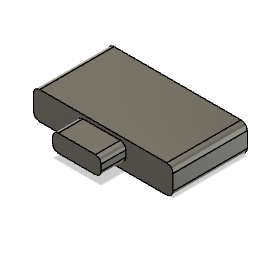
LED retaining Peg v1 (Autodesk Fusion 360 design; units mm, degrees)
Autodesk Fusion 360 part; units mm, degrees
sketch "Sketch1" plane through (0, 0, 0) normal (0, 1, 0) x (1, 0, 0)
  line L0 (14.75, 62.5) -> (-14.75, 62.5)
  line L1 (-14.75, 62.5) -> (-14.75, -62.5)
  line L2 (-14.75, -62.5) -> (14.75, -62.5)
  line L3 (14.75, -62.5) -> (14.75, 62.5)
  line L4 (14.75, 62.5) -> (-14.75, -62.5) construction
  line L5 (-14.75, 62.5) -> (14.75, -62.5) construction
  dimension "d1" = 29.5
  dimension "d4" = 125
  constraint perpendicular L0 L1
  constraint parallel L0 L2
  constraint parallel L1 L3
  constraint horizontal L0
  constraint coincident L4 origin
  constraint coincident L5 origin
  measures "d1" distance of L1.end L2.end
  measures "d4" distance of L0.end L1.end
extrude "Extrude1" add sketch "Sketch1" along normal blind 25 makes body 1
sketch "Sketch2" plane through (14.75, 0, 0) normal (1, 0, 0) x (0, 0, -1)
  line L0 (-62.5, 0) -> (62.5, 0)
  line L1 (62.5, 25) -> (-62.5, 25)
  line L2 (-62.5, 25) -> (-62.5, 0)
  line L3 (-57.5, 0) -> (-41.5, 0)
  line L4 (-41.5, 0) -> (-41.5, 22)
  line L5 (-41.5, 22) -> (-57.5, 22)
  line L6 (-57.5, 22) -> (-57.5, 0)
  dimension "d5" = 16
  dimension "d6" = 5
  dimension "d70" = 3
  constraint horizontal L3
  constraint vertical L4
  constraint horizontal L5
  constraint vertical L6
  constraint coincident L0 L3.start
  measures "d5" distance of L4.end L5.end
  measures "d6" distance of L2 L6
  measures "d70" distance of L1 L5
sketch "Sketch3" plane through (-14.75, 0, 0) normal (-1, 0, 0) x (0, 0, 1)
  line L0 (62.5, 0) -> (62.5, 25)
  line L1 (62.5, 25) -> (-62.5, 25)
  line L2 (-62.5, 25) -> (-62.5, 0)
  line L3 (-62.5, 0) -> (62.5, 0)
  line L4 (-57.5, 0) -> (54.5, 0)
  line L5 (54.5, 0) -> (54.5, 17)
  line L6 (54.5, 17) -> (-57.5, 17)
  line L7 (-57.5, 17) -> (-57.5, 0)
  dimension "d51" = 5
  dimension "d69" = 8
  dimension "d93" = 112
  constraint horizontal L4
  constraint vertical L5
  constraint horizontal L6
  constraint vertical L7
  constraint collinear L3 L4
  measures "d51" distance of L2 L7
  measures "d69" distance of L1 L6
  measures "d93" distance of L5 L7
extrude "Extrude3" cut sketch "Sketch3" against normal blind 26 contours L3 L4 L5 L6 L7 bodies 1
sketch "Sketch4" plane through (-14.75, 0, 0) normal (-1, 0, 0) x (0, 0, 1)
  line L0 (54.5, 17) -> (54.5, 0)
  line L1 (54.5, 0) -> (62.5, 0)
  line L2 (62.5, 0) -> (62.5, 25)
  line L3 (62.5, 25) -> (-62.5, 25)
  line L4 (-62.5, 25) -> (-62.5, 0)
  line L5 (-62.5, 0) -> (-57.5, 0)
  line L6 (-57.5, 17) -> (54.5, 17)
  line L7 (-54.0622, 25) -> (-48, 21.5)
  line L8 (-48, 21.5) -> (37, 21.5)
  line L9 (37, 21.5) -> (43.0622, 25)
  line L10 (-57.5, 0) -> (-57.5, 17)
  dimension "d16" = 3.5
  dimension "d44" = 150
  dimension "d45" = 150
  dimension "d46" = 85
  dimension "d116" = 14.5
  constraint coincident L3 L7.start
  constraint parallel L3 L8
  constraint coincident L3 L9.end
  measures "d16" vertical distance of L7.start L7.end
  measures "d44" angle of L7 L8
  measures "d45" angle of L8 L9
  measures "d46" distance of L7.end L8.end
  measures "d116" distance of L4 L7.end
extrude "Extrude4" cut sketch "Sketch4" against normal through all contours L3 L7 L8 L9 bodies 1
sketch "Sketch5" plane through (-14.75, 0, 0) normal (-1, 0, 0) x (0, 0, 1)
  line L0 (43.0622, 25) -> (37, 21.5)
  line L1 (37, 21.5) -> (-48, 21.5)
  line L2 (-48, 21.5) -> (-54.0622, 25)
  line L3 (-62.5, 25) -> (-62.5, 0)
  line L4 (-62.5, 0) -> (-57.5, 0)
  line L5 (-57.5, 17) -> (54.5, 17)
  line L6 (54.5, 17) -> (54.5, 0)
  line L7 (54.5, 0) -> (62.5, 0)
  line L8 (-53, 21.5) -> (50.5, 21.5)
  line L9 (50.5, 21.5) -> (50.5, 18.55)
  line L10 (50.5, 18.55) -> (-53, 18.55)
  line L11 (-53, 18.55) -> (-53, 21.5)
  line L12 (-57.5, 0) -> (-57.5, 17)
  line L13 (62.5, 0) -> (62.5, 25)
  line L14 (-54.0622, 25) -> (-62.5, 25)
  line L15 (62.5, 25) -> (43.0622, 25)
  dimension "d22" = 2.95
  dimension "d48" = 13.5
  dimension "d107" = 5
  constraint horizontal L8
  constraint vertical L9
  constraint horizontal L10
  constraint vertical L11
  constraint collinear L1 L8
  measures "d22" distance of L8.start L10.end
  measures "d48" distance of L0.end L8.end
  measures "d107" distance of L1.end L8.start
extrude "Extrude5" cut sketch "Sketch5" against normal blind 26 contours L1 L8 L9 L10 L11 bodies 1
sketch "Sketch14" plane through (-14.75, 0, 0) normal (-1, 0, 0) x (0, 0, 1)
  line L0 (37, 21.5) -> (50.5, 21.5)
  line L1 (50.5, 21.5) -> (50.5, 18.55)
  line L2 (50.5, 18.55) -> (-53, 18.55)
  line L3 (-53, 18.55) -> (-53, 21.5)
  line L4 (-48, 21.5) -> (-54.0622, 25)
  line L5 (-54.0622, 25) -> (-62.5, 25)
  line L6 (-62.5, 25) -> (-62.5, 0)
  line L7 (-62.5, 0) -> (-57.5, 0)
  line L8 (-57.5, 0) -> (-57.5, 17)
  line L9 (-57.5, 17) -> (54.5, 17)
  line L10 (54.5, 17) -> (54.5, 0)
  line L11 (54.5, 0) -> (62.5, 0)
  line L12 (62.5, 0) -> (62.5, 25)
  line L13 (62.5, 25) -> (43.0622, 25)
  line L14 (43.0622, 25) -> (37, 21.5)
  line L15 (-53, 21.5) -> (50.5, 21.5)
  line L16 (50.5, 21.5) -> (50.5, 21.75)
  line L17 (50.5, 21.75) -> (-53, 21.75)
  line L18 (-53, 21.75) -> (-53, 21.5)
  line L19 (-53, 21.5) -> (-48, 21.5)
  dimension "d90" = 0.25
  constraint horizontal L15
  constraint vertical L16
  constraint horizontal L17
  constraint vertical L18
  constraint coincident L3.end L15.start
  constraint collinear L1 L16
  measures "d90" distance of L15 L17
extrude "Extrude14" cut sketch "Sketch14" against normal up to surface (26 mm away) contours L0 L14 L15 L16 L17 | L4 L15 L17 L18 L19 bodies 1
ref_plane "WorkPlane1" through (0, 12.5, 0) normal (0, 0, -1) x (-1, 0, 0)
sketch "Sketch6" plane through (0, 0, -62.5) normal (0, 0, -1) x (-1, 0, 0)
  line L0 (-14.75, 0) -> (14.75, 0)
  line L1 (14.75, 0) -> (14.75, 25)
  line L2 (-14.75, 25) -> (-14.75, 0)
  line L3 (14.75, 25) -> (-14.75, 25)
  line L4 (14.75, 17) -> (14.75, 8)
  line L5 (14.75, 8) -> (17.75, 8)
  line L6 (17.75, 8) -> (17.75, 17)
  line L7 (17.75, 17) -> (14.75, 17)
  line L8 (17.75, 12.5) -> (14.75, 12.5) construction
  dimension "d52" = 8
  dimension "d53" = 8
  dimension "d54" = 3
  constraint coincident L1 L4.start
  constraint coincident L1 L4.end
  constraint perpendicular L3 L4
  constraint parallel L1 L6
  constraint midpoint L6 L8.start
  constraint midpoint L4 L8.end
  constraint horizontal L8
  constraint horizontal L7
  measures "d52" distance of L0 L4.end
  measures "d53" distance of L3 L4.start
  measures "d54" distance of L4 L6
sketch "Sketch7" plane through (0, 0, -62.5) normal (0, 0, -1) x (-1, 0, 0)
  line L0 (14.75, 0) -> (-14.75, 0)
  line L1 (-14.75, 0) -> (-14.75, 25)
  line L2 (-14.75, 17) -> (-14.75, 8)
  line L3 (-14.75, 8) -> (-11.75, 8)
  line L4 (-14.75, 17) -> (-11.75, 17)
  line L5 (-11.75, 17) -> (-11.75, 8)
  line L6 (-11.75, 12.5) -> (-14.75, 12.5) construction
  dimension "d56" = 8
  dimension "d57" = 8
  dimension "d58" = 3
  constraint coincident L1 L2.start
  constraint coincident L1 L2.end
  constraint midpoint L5 L6.start
  constraint midpoint L2 L6.end
  constraint horizontal L6
  constraint horizontal L4
  measures "d56" distance of L0.end L2.end
  measures "d57" distance of L1.end L2.start
  measures "d58" distance of L2 L5
extrude "Extrude6" add sketch "Sketch6" against normal blind 5 contours L1 L4 L5 L6 L7 bodies 1
extrude "Extrude7" cut sketch "Sketch7" against normal blind 5.5 bodies 1
mirror "Mirror1" about plane through (0, 12.5, 0) normal (0, 0, -1) of "Extrude6", "Extrude7"
sketch "Sketch10" plane through (0, 0, -62.5) normal (0, 0, -1) x (-1, 0, 0)
  line L0 (-11.75, 8) -> (-14.75, 8)
  line L1 (-14.75, 8) -> (-14.75, 0)
  line L2 (-14.75, 0) -> (14.75, 0)
  line L3 (14.75, 0) -> (14.75, 8)
  line L4 (14.75, 8) -> (17.75, 8)
  line L5 (17.75, 8) -> (17.75, 17)
  line L6 (17.75, 17) -> (14.75, 17)
  line L7 (14.75, 17) -> (14.75, 25)
  line L8 (14.75, 25) -> (-14.75, 25)
  line L9 (-14.75, 25) -> (-14.75, 17)
  line L10 (-14.75, 17) -> (-11.75, 17)
  line L11 (-11.75, 17) -> (-11.75, 8)
  circle A0 centre (1.75, 8) radius 2
  line L12 (14.75, 17) -> (-11.25, 17)
  line L13 (1.75, 8) -> (1.75, 17) construction
  dimension "d60" = 4
  dimension "d61" = 8
  constraint coincident A0.centre L13.start
  constraint midpoint L12 L13.end
  constraint perpendicular L12 L13
  measures "d60" diameter of A0
  measures "d61" distance of L2 A0.centre
extrude "Extrude10" cut sketch "Sketch10" against normal blind 5 contours A0 bodies 1
sketch "Sketch12" plane through (14.75, 0, 0) normal (1, 0, 0) x (0, 0, -1)
  line L0 (-62.5, 17) -> (-57, 17)
  line L1 (-62.5, 0) -> (62.5, 0)
  line L2 (62.5, 0) -> (62.5, 8)
  line L3 (62.5, 8) -> (57, 8)
  line L4 (57, 8) -> (57, 17)
  line L5 (57, 17) -> (62.5, 17)
  line L6 (62.5, 17) -> (62.5, 25)
  line L7 (62.5, 25) -> (54.0622, 25)
  line L8 (54.0622, 25) -> (48, 21.5)
  line L9 (48, 21.5) -> (-37, 21.5)
  line L10 (-37, 21.5) -> (-43.0622, 25)
  line L11 (-43.0622, 25) -> (-62.5, 25)
  line L12 (-62.5, 8) -> (-62.5, 0)
  line L13 (-41.5, 18.5) -> (-45, 22)
  line L14 (-57, 17) -> (-57, 8)
  line L15 (-57, 8) -> (-62.5, 8)
  line L16 (-62.5, 25) -> (-62.5, 17)
sketch "Sketch13" plane through (0, 0, 62.5) normal (0, 0, 1) x (1, 0, 0)
  line L0 (14.75, 8) -> (11.75, 8)
  line L1 (11.75, 8) -> (11.75, 17)
  line L2 (11.75, 17) -> (14.75, 17)
  line L3 (14.75, 17) -> (14.75, 25)
  line L4 (14.75, 25) -> (-14.75, 25)
  line L5 (-14.75, 25) -> (-14.75, 17)
  line L6 (-14.75, 17) -> (-17.75, 17)
  line L7 (-17.75, 17) -> (-17.75, 8)
  line L8 (-17.75, 8) -> (-14.75, 8)
  line L9 (-14.75, 8) -> (-14.75, 0)
  line L10 (-14.75, 0) -> (14.75, 0)
  line L11 (14.75, 0) -> (14.75, 8)
  line L12 (14.75, 17.4) -> (11.35, 17.4)
  line L13 (11.35, 17.4) -> (11.35, 7.6)
  line L14 (11.35, 7.6) -> (14.75, 7.6)
  dimension "d83" = 0.4
  dimension "d84" = 0.4
  dimension "d85" = 0.4
  constraint coincident L3 L12.start
  constraint parallel L1 L13
  constraint coincident L11 L14.end
  constraint parallel L0 L14
  constraint parallel L2 L12
  measures "d83" distance of L2 L12
  measures "d84" distance of L0 L14
  measures "d85" distance of L1 L13
extrude "Extrude13" cut sketch "Sketch13" against normal blind 5.5 contours L0 L1 L2 L3 L11 L12 L13 L14 bodies 1
mirror "Mirror2" about plane through (0, 0, 0) normal (0, 0, 1) of "Extrude13"
sketch "Sketch15" plane through (0, 17, 0) normal (0, -1, 0) x (1, 0, 0)
  line L0 (-14.75, 54.5) -> (-14.75, -57.5)
  line L1 (-14.75, -57.5) -> (11.25, -57.5)
  line L2 (11.25, -57.5) -> (11.25, 54.5)
  line L3 (11.25, 54.5) -> (-14.75, 54.5)
  line L4 (11.25, 50.5) -> (-14.75, 50.5) construction
  line L5 (-4.75, 51.5) -> (1.25, 51.5)
  line L6 (1.25, 51.5) -> (1.25, 45.5)
  line L7 (1.25, 45.5) -> (-4.75, 45.5)
  line L8 (-4.75, 45.5) -> (-4.75, 51.5)
  line L9 (-4.75, 50) -> (-6.95, 50)
  line L10 (-6.95, 50) -> (-6.95, 47)
  line L11 (-6.95, 47) -> (-4.75, 47)
  line L12 (-4.75, 47) -> (-4.75, 50)
  line L13 (1.25, 50) -> (3.45, 50)
  line L14 (3.45, 50) -> (3.45, 47)
  line L15 (3.45, 47) -> (1.25, 47)
  line L16 (1.25, 47) -> (1.25, 50)
  line L17 (-14.75, 50.5) -> (11.25, 50.5)
  line L18 (-1.75, 50.5) -> (-1.75, 51.5) construction
  dimension "d94" = 6
  dimension "d95" = 6
  dimension "d96" = 2.2
  dimension "d97" = 3
  dimension "d118" = 1
  constraint horizontal L5
  constraint vertical L6
  constraint horizontal L7
  constraint vertical L8
  constraint horizontal L9
  constraint vertical L10
  constraint horizontal L11
  constraint vertical L12
  constraint coincident L8 L9.start
  constraint horizontal L13
  constraint vertical L14
  constraint horizontal L15
  constraint vertical L16
  constraint coincident L6 L13.start
  constraint midpoint L8 L12
  constraint midpoint L6 L16
  constraint equal L9 L13
  constraint equal L10 L14
  constraint midpoint L4 L18.start
  constraint midpoint L5 L18.end
  constraint vertical L18
  measures "d94" distance of L5.start L5.end
  measures "d95" distance of L5.start L7.end
  measures "d96" distance of L9.start L9.end
  measures "d97" distance of L9.end L10.end
  measures "d118" distance of L4 L5
extrude "Extrude15" cut sketch "Sketch15" against normal up to surface (4.75 mm away) contours L6 L7 L8 L12 L16 L17 | L5 L6 L8 L17 | L8 L9 L10 L11 L12 | L6 L13 L14 L15 L16 bodies 1
sketch "Sketch17" plane through (-14.75, 0, 0) normal (-1, 0, 0) x (0, 0, 1)
  line L0 (57.5, 17) -> (62.5, 17)
  line L1 (62.5, 17) -> (62.5, 25)
  line L2 (62.5, 25) -> (43.0622, 25)
  line L3 (43.0622, 25) -> (37.433, 21.75)
  line L4 (37.433, 21.75) -> (50.5, 21.75)
  line L5 (50.5, 21.75) -> (50.5, 18.55)
  line L6 (50.5, 18.55) -> (-53, 18.55)
  line L7 (-53, 18.55) -> (-53, 21.75)
  line L8 (-53, 21.75) -> (-48.433, 21.75)
  line L9 (-48.433, 21.75) -> (-54.0622, 25)
  line L10 (-54.0622, 25) -> (-62.5, 25)
  line L11 (-62.5, 25) -> (-62.5, 17)
  line L12 (-62.5, 17) -> (-57.5, 17)
  line L13 (-57.5, 17) -> (54.5, 17)
  line L14 (54.5, 17) -> (54.5, 0)
  line L15 (-57.9, 23.5125) -> (54.9, 23.5125)
  line L16 (54.9, 23.5125) -> (54.9, 20.9313)
  line L17 (54.9, 20.9313) -> (-57.9, 20.9313)
  line L18 (-57.9, 20.9313) -> (-57.9, 23.5125)
  line L19 (62.5, 8) -> (57.5, 8)
  line L20 (57.5, 8) -> (57.5, 17)
  line L21 (54.5, 0) -> (62.5, 0)
  line L22 (62.5, 0) -> (62.5, 8)
  dimension "d109" = 2.3813
  dimension "d110" = 2.5812
  dimension "d111" = 4.6
  dimension "d115" = 112.8
  constraint horizontal L15
  constraint vertical L16
  constraint horizontal L17
  constraint vertical L18
  constraint coincident L16.end L17.start
  measures "d109" distance of L6 L17
  measures "d110" distance of L15.start L17.end
  measures "d111" distance of L11 L18
  measures "d115" distance of L15.start L15.end
extrude "Extrude17" cut sketch "Sketch17" against normal blind 30 contours L3 L4 L5 L15 L16 L17 | L3 L4 L5 L7 L8 L9 L15 L17 | L7 L8 L9 L15 L17 L18 bodies 1
sketch "Sketch18" plane through (11.25, 0, 0) normal (-1, 0, 0) x (0, 0, 1)
  line L0 (-57.5, 17) -> (-57.5, 0)
  line L1 (-57.5, 0) -> (54.5, 0)
  line L2 (54.5, 0) -> (54.5, 17)
  line L3 (54.5, 17) -> (-57.5, 17)
  line L4 (42.5, 17) -> (54.5, 17)
  line L5 (54.5, 17) -> (54.5, 0)
  line L6 (54.5, 0) -> (42.5, 0)
  line L7 (42.5, 0) -> (42.5, 17)
  line L8 (50, 17) -> (47, 17)
  line L9 (48.5, 17) -> (48.5, 0) construction
  dimension "d117" = 12
  constraint horizontal L4
  constraint vertical L5
  constraint horizontal L6
  constraint vertical L7
  constraint coincident L1 L2.start
  constraint coincident L3 L4.start
  constraint midpoint L6 L9.end
  constraint coincident L8 L9.start
  constraint vertical L9
  constraint midpoint L8 L9.start
  measures "d117" distance of L1.end L6.end
extrude "Extrude18" cut sketch "Sketch18" against normal through all contours L1 L2 L3 L4 L5 L6 L7 L8 bodies 1
fillet "Fillet5" radius 1 4 edges at (-6.95, 17.775, 50) (-6.95, 17.775, 47) (3.45, 17.775, 47) (3.45, 17.775, 50) on bodies 1
sketch "Sketch19" plane through (11.25, 0, 0) normal (-1, 0, 0) x (0, 0, 1)
  line L0 (50.5, 20.9313) -> (-53, 20.9313)
  line L1 (-53, 20.9313) -> (-53, 18.55)
  line L2 (-53, 18.55) -> (50.5, 18.55)
  line L3 (50.5, 18.55) -> (50.5, 20.9313)
  line L4 (-53, 20.9313) -> (50.5, 20.9313)
  line L5 (50.5, 20.9313) -> (50.5, 20.8813)
  line L6 (50.5, 20.8813) -> (-53, 20.8813)
  line L7 (-53, 20.8813) -> (-53, 20.9313)
  constraint horizontal L4
  constraint vertical L5
  constraint horizontal L6
  constraint vertical L7
  constraint coincident L3 L5.end
  constraint coincident L0.end L1.start
extrude "Extrude19" cut sketch "Sketch19" against normal through all contours L0 L1 L3 L4 L5 L6 L7 bodies 1
sketch "Sketch20" plane through (0, 17, 0) normal (0, -1, 0) x (1, 0, 0)
  line L0 (1.25, 50) -> (2.45, 50)
  arc A0 (3.45, 49) -> (2.45, 50) centre (2.45, 49) ccw
  line L1 (3.45, 49) -> (3.45, 48)
  arc A1 (2.45, 47) -> (3.45, 48) centre (2.45, 48) ccw
  line L2 (2.45, 47) -> (1.25, 47)
  line L3 (1.25, 47) -> (1.25, 45.5)
  line L4 (1.25, 45.5) -> (-4.75, 45.5)
  line L5 (-4.75, 45.5) -> (-4.75, 47)
  line L6 (-4.75, 47) -> (-5.95, 47)
  arc A2 (-6.95, 48) -> (-5.95, 47) centre (-5.95, 48) ccw
  line L7 (-6.95, 48) -> (-6.95, 49)
  arc A3 (-5.95, 50) -> (-6.95, 49) centre (-5.95, 49) ccw
  line L8 (-5.95, 50) -> (-4.75, 50)
  line L9 (-4.75, 50) -> (-4.75, 51.5)
  line L10 (-4.75, 51.5) -> (1.25, 51.5)
  line L11 (1.25, 51.5) -> (1.25, 50)
  line L12 (-14.75, 54.5) -> (-14.75, -57.5)
  line L13 (-14.75, -57.5) -> (11.25, -57.5)
  line L14 (11.25, -57.5) -> (11.25, 42.5)
  line L15 (11.25, 42.5) -> (14.75, 42.5)
  line L16 (14.75, 42.5) -> (14.75, 54.5)
  line L17 (14.75, 54.5) -> (-14.75, 54.5)
  line L18 (11.25, 42.5) -> (-14.75, 42.5)
  constraint coincident L14.end L15.start
  constraint coincident L12 L18.end
  constraint perpendicular L12 L18
extrude "Extrude20" add sketch "Sketch20" along normal blind 0.5 contours L12 L15 L16 L17 L18 bodies 1
sketch "Sketch21" plane through (14.75, 0, 0) normal (1, 0, 0) x (0, 0, -1)
  line L0 (-50.5, 20.8813) -> (-50.5, 20.9313)
  line L1 (-50.5, 20.9313) -> (-54.9, 20.9313)
  line L2 (-54.9, 20.9313) -> (-54.9, 23.5125)
  line L3 (-54.9, 23.5125) -> (-40.4858, 23.5125)
  line L4 (-40.4858, 23.5125) -> (-43.0622, 25)
  line L5 (-43.0622, 25) -> (-62.5, 25)
  line L6 (-62.5, 25) -> (-62.5, 17.4)
  line L7 (-62.5, 17.4) -> (-57, 17.4)
  line L8 (-57, 17.4) -> (-57, 7.6)
  line L9 (-57, 7.6) -> (-62.5, 7.6)
  line L10 (-62.5, 7.6) -> (-62.5, 0)
  line L11 (-62.5, 0) -> (-54.5, 0)
  line L12 (-54.5, 0) -> (-54.5, 16.5)
  line L13 (-54.5, 16.5) -> (-42.5, 16.5)
  line L14 (-42.5, 16.5) -> (-42.5, 0)
  line L15 (-42.5, 0) -> (62.5, 0)
  line L16 (62.5, 0) -> (62.5, 7.6)
  line L17 (62.5, 7.6) -> (57, 7.6)
  line L18 (57, 7.6) -> (57, 17.4)
  line L19 (57, 17.4) -> (62.5, 17.4)
  line L20 (62.5, 17.4) -> (62.5, 25)
  line L21 (62.5, 25) -> (54.0622, 25)
  line L22 (54.0622, 25) -> (51.4858, 23.5125)
  line L23 (51.4858, 23.5125) -> (57.9, 23.5125)
  line L24 (57.9, 23.5125) -> (57.9, 20.9313)
  line L25 (57.9, 20.9313) -> (53, 20.9313)
  line L26 (53, 20.9313) -> (53, 20.8813)
  line L27 (53, 20.8813) -> (-50.5, 20.8813)
  line L28 (-54.5, 14.5) -> (-52.5, 16.5)
  line L29 (-42.5, 14.5) -> (-44.5, 16.5)
  dimension "d125" = 2
  dimension "d126" = 2
  dimension "d127" = 2
  constraint coincident L12 L28.start
  constraint coincident L13 L28.end
  constraint coincident L14 L29.start
  constraint coincident L13 L29.end
  constraint perpendicular L28 L29
  measures "d125" distance of L12.end L28.end
  measures "d126" distance of L14 L29.end
  measures "d127" distance of L13 L29.start
extrude "Extrude21" add sketch "Sketch21" against normal up to surface (3.5 mm away) contours L12 L13 L28 | L13 L14 L29 bodies 1
sketch "Sketch22" plane through (0, 0, 54.5) normal (0, 0, -1) x (-1, 0, 0)
  line L0 (-11.25, 14.5) -> (-14.75, 14.5)
  line L1 (-14.75, 14.5) -> (-14.75, 0)
  line L2 (-14.75, 0) -> (14.75, 0)
  line L3 (14.75, 0) -> (14.75, 16.5)
  line L4 (14.75, 16.5) -> (-11.25, 16.5)
  line L5 (-11.25, 16.5) -> (-11.25, 14.5)
  line L6 (-2.25, 15.5) -> (5.75, 15.5)
  line L7 (5.75, 15.5) -> (5.75, 12.5)
  line L8 (5.75, 12.5) -> (-2.25, 12.5)
  line L9 (-2.25, 12.5) -> (-2.25, 15.5)
  line L10 (1.75, 16.5) -> (1.75, 15.5) construction
  dimension "d130" = 3
  dimension "d131" = 8
  dimension "d132" = 1
  constraint horizontal L6
  constraint vertical L7
  constraint horizontal L8
  constraint vertical L9
  constraint midpoint L4 L10.start
  constraint midpoint L6 L10.end
  constraint vertical L10
  measures "d130" distance of L6.start L8.end
  measures "d131" distance of L7.end L8.end
  measures "d132" distance of L4 L6
extrude "Extrude22" cut sketch "Sketch22" against normal blind 4 contours L6 L7 L8 L9 bodies 1
fillet "Fillet6" radius 1 4 edges at (2.25, 15.5, 56.5) (2.25, 12.5, 56.5) (-5.75, 12.5, 56.5) (-5.75, 15.5, 56.5) on bodies 1
sketch "Sketch23" plane through (0, 16.5, 0) normal (0, -1, 0) x (1, 0, 0)
  line L0 (11.25, 44.5) -> (14.75, 44.5)
  line L1 (14.75, 44.5) -> (14.75, 52.5)
  line L2 (14.75, 52.5) -> (11.25, 52.5)
  line L3 (11.25, 52.5) -> (11.25, 54.5)
  line L4 (11.25, 54.5) -> (-14.75, 54.5)
  line L5 (-14.75, 54.5) -> (-14.75, 42.5)
  line L6 (-14.75, 42.5) -> (11.25, 42.5)
  line L7 (11.25, 42.5) -> (11.25, 44.5)
  arc A0 (-5.95, 50) -> (-6.95, 49) centre (-5.95, 49) ccw
  line L8 (-5.95, 50) -> (-4.75, 50)
  line L9 (-4.75, 50) -> (-4.75, 51.5)
  line L10 (-4.75, 51.5) -> (1.25, 51.5)
  line L11 (1.25, 51.5) -> (1.25, 50)
  line L12 (1.25, 50) -> (2.45, 50)
  arc A1 (3.45, 49) -> (2.45, 50) centre (2.45, 49) ccw
  line L13 (3.45, 49) -> (3.45, 48)
  arc A2 (2.45, 47) -> (3.45, 48) centre (2.45, 48) ccw
  line L14 (2.45, 47) -> (1.25, 47)
  line L15 (1.25, 47) -> (1.25, 45.5)
  line L16 (1.25, 45.5) -> (-4.75, 45.5)
  line L17 (-4.75, 45.5) -> (-4.75, 47)
  line L18 (-4.75, 47) -> (-5.95, 47)
  arc A3 (-6.95, 48) -> (-5.95, 47) centre (-5.95, 48) ccw
  line L19 (-6.95, 48) -> (-6.95, 49)
  line L20 (-14.75, 54.5) -> (11.25, 54.5)
  line L21 (11.25, 54.5) -> (11.25, 42.5)
  line L22 (11.25, 42.5) -> (-14.75, 42.5)
  line L23 (-14.75, 42.5) -> (-14.75, 54.5)
  line L24 (11.25, 54.5) -> (9.75, 54.5) construction
  line L25 (9.75, 54.5) -> (9.75, 42.5)
  line L26 (9.75, 42.5) -> (11.25, 42.5) construction
  line L27 (11.25, 42.5) -> (11.25, 54.5) construction
  line L28 (-14.75, 54.5) -> (-12.75, 54.5) construction
  line L29 (-12.75, 54.5) -> (-12.75, 42.5)
  line L30 (-12.75, 42.5) -> (-14.75, 42.5) construction
  line L31 (-14.75, 42.5) -> (-14.75, 54.5) construction
  dimension "d139" = 1.5
  dimension "d140" = 2
  dimension "d141" = 12
  constraint horizontal L20
  constraint vertical L21
  constraint horizontal L22
  constraint vertical L23
  constraint coincident L6.end L7.start
  constraint coincident L4.end L5.start
  constraint horizontal L24
  constraint vertical L25
  constraint horizontal L26
  constraint vertical L27
  constraint horizontal L28
  constraint vertical L29
  constraint horizontal L30
  constraint vertical L31
  measures "d139" distance of L3.end L24.end
  measures "d140" distance of L4.end L28.end
  measures "d141" distance of L4.end L5.end
sketch "Sketch24" plane through (0, 0, 54.5) normal (0, 0, -1) x (-1, 0, 0)
  line L0 (5.75, 14.5) -> (5.75, 13.5)
  arc A0 (4.75, 12.5) -> (5.75, 13.5) centre (4.75, 13.5) ccw
  line L1 (4.75, 12.5) -> (-1.25, 12.5)
  arc A1 (-2.25, 13.5) -> (-1.25, 12.5) centre (-1.25, 13.5) ccw
  line L2 (-2.25, 13.5) -> (-2.25, 14.5)
  arc A2 (-1.25, 15.5) -> (-2.25, 14.5) centre (-1.25, 14.5) ccw
  line L3 (-1.25, 15.5) -> (4.75, 15.5)
  arc A3 (5.75, 14.5) -> (4.75, 15.5) centre (4.75, 14.5) ccw
  line L4 (-11.25, 14.5) -> (-14.75, 14.5)
  line L5 (-14.75, 14.5) -> (-14.75, 0)
  line L6 (-14.75, 0) -> (14.75, 0)
  line L7 (14.75, 0) -> (14.75, 16.5)
  line L8 (14.75, 16.5) -> (-11.25, 16.5)
  line L9 (-11.25, 16.5) -> (-11.25, 14.5)
  line L10 (5.75, 14) -> (-2.25, 14) construction
  line L11 (6.25, 14.5) -> (6.25, 13.5)
  arc A4 (4.75, 12) -> (6.25, 13.5) centre (4.75, 13.5) ccw
  line L12 (4.75, 12) -> (-1.25, 12)
  arc A5 (-2.75, 13.5) -> (-1.25, 12) centre (-1.25, 13.5) ccw
  line L13 (-2.75, 13.5) -> (-2.75, 14.5)
  arc A6 (-1.25, 16) -> (-2.75, 14.5) centre (-1.25, 14.5) ccw
  line L14 (-1.25, 16) -> (4.75, 16)
  arc A7 (6.25, 14.5) -> (4.75, 16) centre (4.75, 14.5) ccw
  dimension "d136" = 0.5
  constraint midpoint L0 L10.start
  constraint midpoint L2 L10.end
extrude "Extrude23" add sketch "Sketch24" along normal blind 8 separate body contours L0 A0 L1 A1 L2 A2 L3 A3 | L11 A4 L12 A5 L13 A6 L14 A7 makes body 2
extrude "Extrude24" add sketch "Sketch23" along normal blind 5 and the other way blind -0.5 contours L4 L6 L20 L22 L25 L29 | A0 L8 L9 L10 L11 L12 A1 L13 A2 L14 L15 L16 L17 L18 A3 L19 bodies 2
extrude "Extrude25" add sketch "Sketch24" against normal up to surface (4 mm away) separate body contours L0 A0 L1 A1 L2 A2 L3 A3 makes body 3
move_face "OffsetFaces1" offset -0.1 8 faces at (-2.75, 12.5, 55.8333) (-5.3682, 12.7139, 57.1667) (-5.7218, 14.7358, 57.1667) (-0.75, 15.5, 55.8333) (-5.75, 14.1667, 55.8333) (2.2489, 14.5476, 57.1667) (2.25, 13.8333, 55.8333) (2.2218, 13.2642, 57.1667) on bodies 3
combine "Combine1" operation add target body 2 tool bodies 3
fillet "Fillet7" radius 1 4 edges at (-12.75, 16, 48.5) (9.75, 16, 48.5) (-12.75, 11.5, 48.5) (9.75, 11.5, 48.5) on bodies 2
hidden bodies 1
equation "d48 = 12 mm + 1.5 mm"
equation "d109 = ( 3 / 32 ) * 1 in"
equation "d110 = ( 3 / 32 ) * 1 in + 0.2 mm"
equation "d115 = 112 mm + 0.8 mm"
equation "d116 = 9.50 mm + 5 mm"
